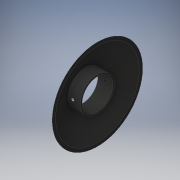
# Autodesk Inventor part: Penahan tanah
Saved by Autodesk Inventor 2019.5 (Build 235369000, 369)
## iProperties
Created: 2022-10-11
Part Number: Penahan tanah
Material: Aluminum 6061-AHC
Document SubType Name: Modeling
Designer: ASUS
Density: 2.7 g/cm^3
Appearance: Aluminum - Dark
Author: ASUS
Autodesk Inventor part; units mm, degrees
ref_plane "YZ Plane" through (0, 0, 0) normal (1, 0, 0) x (0, 1, 0)
ref_plane "XZ Plane" through (0, 0, 0) normal (0, 1, 0) x (-1, 0, 0)
ref_plane "XY Plane" through (0, 0, 0) normal (0, 0, 1) x (1, 0, 0)
sketch "Sketch3" plane through (0, 0, 0) normal (0, 1, 0) x (-1, 0, 0)
  line L0 (0, 0) -> (-30, 0)
  line L1 (-30, 0) -> (-30, -60)
  line L2 (-30, -60) -> (0, 0)
  dimension "d10" = 30
  dimension "d11" = 60
  dimension "d33" = 67.082
  constraints: 6 end point, 1 horizontal, 1 perpendicular
  measures "d10" distance of L0.start L0.end
  measures "d11" distance of L0.end L1.end
  measures "d33" distance of L1.end L0.start
revolve "Revolution4" add sketch "Sketch3" angle 360 about axis through (0, 0, 0) along (1, 0, 0)
sketch "Sketch4" plane through (30, 0, 0) normal (1, 0, 0) x (0, 0, -1)
  point P0 (0, 0)
  point P1 (0, 0)
  constraints: 1 coincident
hole "Hole1" at (30, 0, 0) direction (-1, 0, 0) diameter 41 depth 40.25
shell "Shell2" thickness 2 removed faces 1 at (30, 15.6337, 43.9334)
sketch "Sketch5" plane through (0, 0, 0) normal (0, 0, 1) x (1, 0, 0)
  circle A0 centre (19.9279, 0) radius 1.5
  point P0 (0, 0)
  dimension "d25" = 3
  constraints: 1 centre point
  measures "d25" diameter of A0
extrude "Extrusion1" add sketch "Sketch5" along normal blind 21.5 and the other way blind 24
sketch "Sketch6" plane through (19.9279, 0, -24) normal (0, 0, -1) x (-1, 0, 0)
  point P0 (19.9279, 0)
  point P1 (0.0492, -0.0436)
hole "Hole2" at (19.8787, -0.0436, -24) direction (0, 0, 1) diameter 4 depth 48.25
body "Solid4"
